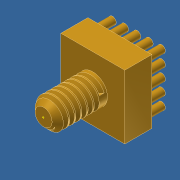
# Autodesk Inventor part: WURTH_7460719_0_8071_J
Saved by Autodesk Inventor 2012 (Build 160160000, 160)
## iProperties
Company: Team 801
Created: 2008-03-31
Part Number: WURTH_7460719_0_8071_J
Document SubType Name: Modeling
Designer: Jeffrey M
Mass: 11.0558 g
Surface Area: 12.9124 cm^2
Volume: 1.30529 cm^3
Density: 8.47 g/cm^3
Material: Brass, Soft Yellow
Catalog Web Link: www.team801.org
Author: Jeffrey M
Autodesk Inventor part; units mm, degrees
ref_plane "YZ Plane" through (0, 0, 0) normal (1, 0, 0) x (0, 1, 0)
ref_plane "XZ Plane" through (0, 0, 0) normal (0, 1, 0) x (-1, 0, 0)
ref_plane "XY Plane" through (0, 0, 0) normal (0, 0, 1) x (1, 0, 0)
sketch "Sketch1" plane through (0, 0, 0) normal (0, 0, 1) x (1, 0, 0)
  line L0 (0, 9.1) -> (0, -9.1) construction
  line L1 (-9.1, 0) -> (9.1, 0) construction
  line L2 (-6.5, 6.5) -> (6.5, 6.5)
  line L3 (6.5, 6.5) -> (6.5, -6.5)
  line L4 (6.5, -6.5) -> (-6.5, -6.5)
  line L5 (-6.5, -6.5) -> (-6.5, 6.5)
  point P0 (0, 0)
  dimension "d0" = 13
  dimension "d1" = 13
  constraints: 8 end point, 2 parallel, 1 horizontal, 1 perpendicular, 2 other
  measures "d0" distance of L4.end L2.start
  measures "d1" distance of L2.start L2.end
extrude "Extrusion1" add sketch "Sketch1" along normal blind 5.5
sketch "Sketch2" plane through (0, 0, 5.5) normal (0, 0, 1) x (1, 0, 0)
  line L0 (0, 9.1) -> (0, -9.1) construction
  line L1 (-9.1, 0) -> (9.1, 0) construction
  circle A0 centre (0, 0) radius 2.975
  dimension "d4" = 5.95
  constraints: 1 centre point, 1 coincident
  measures "d4" diameter of A0
extrude "Extrusion2" add sketch "Sketch2" along normal blind 10
chamfer "Chamfer1" distance 1.25 angle 45 1 edges at (-2.975, 0, 15.5)
sketch "Sketch3" plane through (0, 0, 0) normal (1, 0, 0) x (0, 1, 0)
  line L0 (0, 25.35) -> (0, -4.225) projected
  line L1 (-1.725, 15.5) -> (1.725, 15.5) projected
  line L2 (3, 16) -> (3, 15) construction
  line L3 (3, 15) -> (2.134, 15.5)
  line L4 (2.134, 15.5) -> (3, 16)
  line L5 (2.975, 5.5) -> (2.975, 14.25) projected
  line L6 (2.975, 15.0144) -> (2.975, 15.9856)
  point P0 (0, 0)
  dimension "d10" = 1
  dimension "d11" = 6
  constraints: 8 end point, 3 point on line, 2 equal length, 1 collinear, 1 parallel, 1 perpendicular
  measures "d10" distance of L2.start L2.end
  measures "d11" diameter of L2 L0
coil "Coil1" sketch "Sketch3" operation cut axis through (0, 0, -10) along (0, 0, -1) pitch 1.25 turns 7.2 hand right
sketch "Sketch4" plane through (0, 0, 0) normal (0, 0, -1) x (-1, 0, 0)
  line L0 (0, -9.1) -> (0, 9.1) construction
  line L1 (-9.1, 0) -> (9.1, 0) construction
  circle A0 centre (-5, -5) radius 0.75
  circle A1 centre (-2.5, -5) radius 0.75
  circle A2 centre (0, -5) radius 0.75
  circle A3 centre (2.5, -5) radius 0.75
  circle A4 centre (5, -5) radius 0.75
  circle A5 centre (-5, -2.5) radius 0.75
  circle A6 centre (-2.5, -2.5) radius 0.75
  circle A7 centre (0, -2.5) radius 0.75
  circle A8 centre (2.5, -2.5) radius 0.75
  circle A9 centre (5, -2.5) radius 0.75
  circle A10 centre (-5, 0) radius 0.75
  circle A11 centre (-2.5, 0) radius 0.75
  circle A12 centre (0, 0) radius 0.75
  circle A13 centre (2.5, 0) radius 0.75
  circle A14 centre (5, 0) radius 0.75
  circle A15 centre (-5, 2.5) radius 0.75
  circle A16 centre (-2.5, 2.5) radius 0.75
  circle A17 centre (0, 2.5) radius 0.75
  circle A18 centre (2.5, 2.5) radius 0.75
  circle A19 centre (5, 2.5) radius 0.75
  circle A20 centre (-5, 5) radius 0.75
  circle A21 centre (-2.5, 5) radius 0.75
  circle A22 centre (0, 5) radius 0.75
  circle A23 centre (2.5, 5) radius 0.75
  circle A24 centre (5, 5) radius 0.75
  point P0 (0, 0)
  dimension "d22" = 2.5
  dimension "d25" = 2.5
  dimension "d28" = 1.5
  constraints: 25 centre point, 1 coincident, 1 horizontal, 1 vertical, 48 other
  measures "d22" distance of A0.centre A1.centre
  measures "d25" distance of A0.centre A5.centre
  measures "d28" diameter of A0
extrude "Extrusion3" add sketch "Sketch4" along normal blind 3.5
sketch "Sketch5" plane through (0, 0, 15.5) normal (0, 0, 1) x (1, 0, 0)
  circle A0 centre (0, 0) radius 1.725 projected
body "Solid1"
